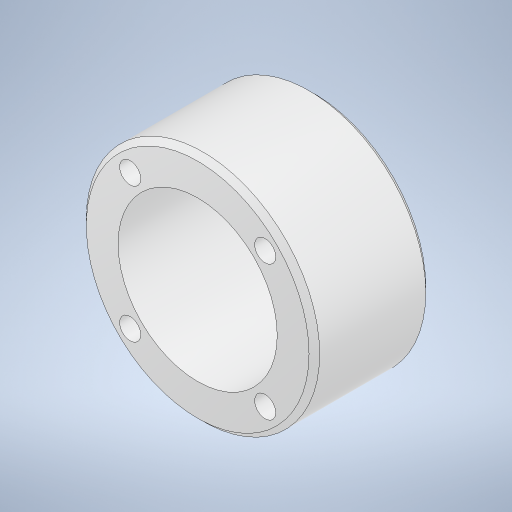
# Autodesk Inventor part: AL Ring
Saved by Autodesk Inventor 2023.2 (Build 272271000, 271)
## iProperties
Created: 2023-05-26
Part Number: AL Ring
Material: Aluminum 6061
Document SubType Name: Modeling
Designer: Nathan Cai
Density: 2.7 g/cm^3
Appearance: Aluminum - Flat
Mass: 5.6683 g
Surface Area: 19.3679 cm^2
Volume: 2.09937 cm^3
Author: Nathan Cai
Autodesk Inventor part; units mm, degrees
ref_plane "YZ Plane" through (0, 0, 0) normal (1, 0, 0) x (0, 1, 0)
ref_plane "XZ Plane" through (0, 0, 0) normal (0, 1, 0) x (-1, 0, 0)
ref_plane "XY Plane" through (0, 0, 0) normal (0, 0, 1) x (1, 0, 0)
sketch "Sketch1" plane through (0, 0, 0) normal (0, 0, 1) x (1, 0, 0)
  circle A0 centre (0, 0) radius 11
  circle A1 centre (0, 0) radius 9 construction
  line L0 (0, 0) -> (0, 11) construction
  line L1 (0, 0) -> (-6.364, 6.364) construction
  circle A2 centre (-6.364, 6.364) radius 1
  circle A3 centre (0, 0) radius 7.5
  circle A4 centre (-6.364, -6.364) radius 1
  circle A5 centre (6.364, -6.364) radius 1
  circle A6 centre (6.364, 6.364) radius 1
  dimension "d0" = 22
  dimension "d1" = 18
  dimension "d2" = 45
  dimension "d3" = 2
  dimension "d4" = 15
  dimension "d7" = 360
  constraints: 5 centre point, 4 coincident, 4 end point, 1 vertical, 1 vertical alignment, 14 other
  measures "d2" angle of L0 L1
  measures "d3" diameter of A2
  measures "d4" diameter of A3
extrude "Extrusion1" add sketch "Sketch1" along normal blind 11
chamfer "Chamfer1" distance 0.5 angle 45 1 edges at (-11, 0, 11)
chamfer "Chamfer2" distance 0.5 angle 45 1 edges at (-11, 0, 0)
sketch "Sketch2" plane through (0, 0, 11) normal (0, 0, 1) x (1, 0, 0)
  line L0 (8, -8) -> (-8, -8)
  line L1 (-8, -8) -> (-8, 8)
  line L2 (-8, 8) -> (8, 8)
  line L3 (8, 8) -> (8, -8)
  line L4 (8, -8) -> (-8, 8) construction
  line L5 (-8, -8) -> (8, 8) construction
  circle A0 centre (0, 0) radius 15
  arc A1 (-6.25, 8) -> (-8, 6.25) centre (-6.25, 6.25) ccw
  arc A2 (-8, -6.25) -> (-6.25, -8) centre (-6.25, -6.25) ccw
  arc A3 (6.25, -8) -> (8, -6.25) centre (6.25, -6.25) ccw
  arc A4 (8, 6.25) -> (6.25, 8) centre (6.25, 6.25) ccw
  point P0 (8, 6.25)
  point P1 (8, -6.25)
  point P2 (6.25, -8)
  point P3 (-6.25, -8)
  point P4 (-8, -6.25)
  point P5 (6.25, 8)
  dimension "d11" = 16
  dimension "d12" = 16
  dimension "d13" = 30
  dimension "d14" = 3.5
  dimension "d17" = 360
  constraints: 12 end point, 8 point on circle, 5 centre point, 3 point on line, 2 midpoint, 2 parallel, 1 coincident, 1 horizontal, 1 perpendicular, 1 tangent, 17 other
  measures "d11" distance of L1.end L2.end
  measures "d12" distance of L0.end L1.end
  measures "d13" diameter of A0
  measures "d14" diameter of A1
body "Solid1"
